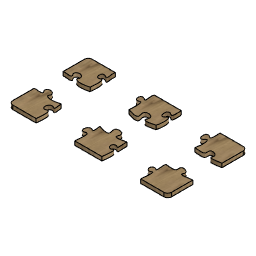
Púslu bretti v2 (Autodesk Fusion 360 design; units mm, degrees)
Autodesk Fusion 360 part; units mm, degrees
sketch "Sketch1" plane through (0, 0, 0) normal (0, 0, 1) x (1, 0, 0)
  line L0 (20, 0) -> (400, 0)
  line L1 (0, 240) -> (0, 20)
  line L2 (400, 260) -> (280, 260)
  line L3 (280, 260) -> (140, 260)
  line L4 (140, 260) -> (20, 260)
  line L5 (420, 240) -> (420, 130)
  line L6 (420, 130) -> (420, 20)
  spline S0 degree 5 poles (420, 130) (416.1569, 129.3347) (408.8145, 128.1) (398.8326, 126.5354) (387.5903, 125.0254) (376.9641, 124.1005) (369.6712, 124.1345) (365.4953, 125.1121) (364.0482, 127) (364.7182, 129.7413) (366.62, 133.2478) (368.5346, 137.3946) (369.2158, 141.9958) (367.694, 146.7817) (363.6047, 151.3716) (357.4467, 155.2591) (350.2289, 157.9216) (343.1844, 158.915) (337.448, 157.9813) (333.7805, 155.1362) (332.1898, 150.8086) (332.0622, 145.7217) (332.5096, 140.6598) (332.6186, 136.2944) (331.8011, 132.9328) (329.8033, 130.5545) (326.5513, 128.9847) (322.0312, 128.048) (316.2309, 127.6288) (309.1523, 127.6444) (300.8011, 128.0454) (293.1087, 128.653) (286.7739, 129.2656) (282.2998, 129.7436) (280, 130) knots 0 0 0 0 0 0 0.033333 0.066667 0.1 0.133333 0.166667 0.2 0.233333 0.266667 0.3 0.333333 0.366667 0.4 0.433333 0.466667 0.5 0.533333 0.566667 0.6 0.633333 0.666667 0.7 0.733333 0.766667 0.8 0.833333 0.866667 0.9 0.933333 0.966667 1 1 1 1 1 1
  spline S1 degree 5 poles (280, 130) (275.8224, 128.8825) (267.8961, 126.843) (257.2935, 124.3707) (245.7371, 122.2512) (235.5527, 121.5576) (229.4432, 122.7719) (226.9787, 125.7728) (227.3955, 130.3359) (229.4779, 136.0973) (231.5057, 142.5292) (231.7666, 149.0092) (228.9911, 154.8796) (222.8666, 159.5099) (214.3976, 162.358) (205.2875, 163.0238) (197.4083, 161.3087) (192.2863, 157.2675) (190.4715, 151.2893) (191.3079, 144.0924) (193.4639, 136.556) (195.2859, 129.5898) (195.2199, 123.9891) (192.1984, 120.2965) (185.5461, 118.8526) (174.8886, 119.8432) (163.0301, 122.6449) (152.2476, 125.8819) (144.2221, 128.5434) (140, 130) knots 0 0 0 0 0 0 0.04 0.08 0.12 0.16 0.2 0.24 0.28 0.32 0.36 0.4 0.44 0.48 0.52 0.56 0.6 0.64 0.68 0.72 0.76 0.8 0.84 0.88 0.92 0.96 1 1 1 1 1 1
  spline S2 degree 5 poles (0, 130) (0.6726, 130.1303) (2.0368, 130.3625) (4.1406, 130.6262) (7.0605, 130.808) (10.8974, 130.7621) (14.9065, 130.4737) (19.0576, 130.005) (23.2997, 129.4607) (27.5558, 128.9989) (31.712, 128.7955) (35.6093, 129.0115) (39.0309, 129.7574) (41.6968, 131.0621) (43.242, 132.8313) (43.385, 134.9274) (42.1144, 137.2617) (39.8723, 139.8827) (37.3749, 142.897) (35.4219, 146.3814) (34.7244, 150.3097) (35.6898, 154.4468) (38.3617, 158.3555) (42.5273, 161.5252) (47.7801, 163.4671) (53.6005, 163.8256) (59.4268, 162.4764) (64.7331, 159.6498) (69.0714, 155.8267) (72.1104, 151.6033) (73.6742, 147.5681) (73.7844, 144.1721) (72.6966, 141.607) (70.9513, 139.6629) (69.2082, 137.9334) (68.0891, 136.0141) (67.978, 133.7535) (69.0147, 131.2602) (71.2092, 128.7604) (74.5314, 126.4828) (78.963, 124.5976) (84.4839, 123.2388) (91.078, 122.5032) (98.7311, 122.4588) (107.4319, 123.1487) (117.1713, 124.5977) (125.7887, 126.3726) (132.7145, 128.0513) (137.5372, 129.3247) (140, 130) knots 0 0 0 0 0 0 0.022222 0.044444 0.066667 0.088889 0.111111 0.133333 0.155556 0.177778 0.2 0.222222 0.244444 0.266667 0.288889 0.311111 0.333333 0.355556 0.377778 0.4 0.422222 0.444444 0.466667 0.488889 0.511111 0.533333 0.555556 0.577778 0.6 0.622222 0.644444 0.666667 0.688889 0.711111 0.733333 0.755556 0.777778 0.8 0.822222 0.844444 0.866667 0.888889 0.911111 0.933333 0.955556 0.977778 1 1 1 1 1 1
  spline S3 degree 5 poles (280, 260) (280.191, 256.8907) (280.5235, 250.9394) (280.8735, 242.8142) (281.042, 233.5862) (280.7527, 224.7165) (279.9574, 218.457) (278.6472, 214.6822) (276.8095, 213.1654) (274.4294, 213.5546) (271.4855, 215.3325) (267.9643, 217.8215) (263.9195, 220.2718) (259.5123, 221.9338) (255.0824, 222.1325) (251.1161, 220.3585) (248.107, 216.3963) (246.4574, 210.4182) (246.3361, 203.1543) (247.6759, 195.7591) (250.2541, 189.4958) (253.7478, 185.4653) (257.7961, 184.3396) (262.0648, 186.0375) (266.2937, 189.5848) (270.2827, 193.5755) (273.8891, 196.5474) (277.02, 197.3547) (279.6286, 195.6325) (281.7019, 191.6447) (283.2467, 185.9595) (284.276, 179.1424) (284.7999, 171.5914) (284.8281, 163.5991) (284.3685, 155.3565) (283.4276, 146.9795) (282.2934, 140.2164) (281.2296, 135.1183) (280.4256, 131.708) (280, 130) knots 0 0 0 0 0 0 0.028571 0.057143 0.085714 0.114286 0.142857 0.171429 0.2 0.228571 0.257143 0.285714 0.314286 0.342857 0.371429 0.4 0.428571 0.457143 0.485714 0.514286 0.542857 0.571429 0.6 0.628571 0.657143 0.685714 0.714286 0.742857 0.771429 0.8 0.828571 0.857143 0.885714 0.914286 0.942857 0.971429 1 1 1 1 1 1
  spline S4 degree 5 poles (280, 130) (279.893, 129.6992) (279.7025, 128.9631) (279.4868, 127.4558) (279.3397, 124.6386) (279.3831, 119.8124) (279.631, 113.8173) (280.0368, 106.9315) (280.5206, 99.6325) (280.9623, 92.629) (281.2121, 86.6861) (281.0987, 82.4762) (280.4373, 80.4102) (279.042, 80.4986) (276.723, 82.1374) (273.3748, 84.3371) (269.0681, 86.0447) (264.1813, 86.486) (259.365, 85.297) (255.346, 82.4331) (252.7746, 78.1432) (252.058, 72.9178) (253.1887, 67.4537) (255.8568, 62.513) (259.5736, 58.7828) (263.7905, 56.7322) (268.0188, 56.4712) (271.9496, 57.6043) (275.4114, 59.408) (278.3264, 61.0095) (280.6676, 61.564) (282.4165, 60.431) (283.562, 57.1434) (284.0982, 51.3798) (284.0237, 42.937) (283.3393, 31.7027) (282.306, 20.4445) (281.2587, 10.7197) (280.4397, 3.668) (280, 0) knots 0 0 0 0 0 0 0.028571 0.057143 0.085714 0.114286 0.142857 0.171429 0.2 0.228571 0.257143 0.285714 0.314286 0.342857 0.371429 0.4 0.428571 0.457143 0.485714 0.514286 0.542857 0.571429 0.6 0.628571 0.657143 0.685714 0.714286 0.742857 0.771429 0.8 0.828571 0.857143 0.885714 0.914286 0.942857 0.971429 1 1 1 1 1 1
  spline S5 degree 5 poles (140, 260) (139.786, 259.149) (139.3949, 257.4189) (138.9194, 254.7391) (138.5076, 250.9966) (138.3554, 246.0496) (138.5404, 240.8764) (139.0108, 235.562) (139.6777, 230.2517) (140.4088, 225.1603) (141.0118, 220.6004) (141.2554, 216.9394) (140.9216, 214.4967) (139.8454, 213.4649) (137.9674, 213.805) (135.3596, 215.2012) (132.1765, 217.1928) (128.6213, 219.2678) (124.9018, 220.9885) (121.2137, 222.0296) (117.7406, 222.1651) (114.6502, 221.2708) (112.0908, 219.3206) (110.188, 216.3856) (109.039, 212.6276) (108.7059, 208.2939) (109.21, 203.7089) (110.5242, 199.275) (112.5703, 195.4454) (115.2295, 192.6298) (118.3503, 191.1054) (121.7572, 190.9403) (125.2582, 191.8765) (128.6582, 193.3586) (131.7822, 194.721) (134.4936, 195.3279) (136.7176, 194.743) (138.4568, 192.857) (139.7601, 189.7597) (140.6986, 185.6454) (141.3343, 180.6897) (141.7144, 175.0249) (141.8752, 168.7528) (141.8426, 161.9461) (141.6342, 154.6547) (141.261, 146.9088) (140.8351, 140.3614) (140.445, 135.2563) (140.1536, 131.7665) (140, 130) knots 0 0 0 0 0 0 0.022222 0.044444 0.066667 0.088889 0.111111 0.133333 0.155556 0.177778 0.2 0.222222 0.244444 0.266667 0.288889 0.311111 0.333333 0.355556 0.377778 0.4 0.422222 0.444444 0.466667 0.488889 0.511111 0.533333 0.555556 0.577778 0.6 0.622222 0.644444 0.666667 0.688889 0.711111 0.733333 0.755556 0.777778 0.8 0.822222 0.844444 0.866667 0.888889 0.911111 0.933333 0.955556 0.977778 1 1 1 1 1 1
  spline S6 degree 5 poles (140, 130) (140.3543, 127.5224) (141.0103, 122.7786) (141.836, 116.2971) (142.6203, 108.9248) (143.0716, 101.8141) (142.9936, 96.7592) (142.3884, 93.6536) (141.2613, 92.3088) (139.623, 92.4356) (137.4899, 93.6129) (134.8881, 95.293) (131.8674, 96.9199) (128.5115, 98.0179) (124.9543, 98.3121) (121.3675, 97.7073) (117.9388, 96.2219) (114.8545, 93.9421) (112.2772, 90.956) (110.3371, 87.3448) (109.1319, 83.2198) (108.7254, 78.7506) (109.1458, 74.1891) (110.3839, 69.9148) (112.3917, 66.3689) (115.0791, 63.9342) (118.3123, 62.8384) (121.9097, 63.0328) (125.6443, 64.1245) (129.2811, 65.5407) (132.6101, 66.6645) (135.4787, 66.9724) (137.8318, 66.1957) (139.6859, 64.2641) (141.0921, 61.2114) (142.0979, 57.0823) (142.7393, 51.9103) (143.0449, 45.725) (143.0355, 38.5494) (142.7258, 30.4016) (142.1253, 21.2949) (141.4167, 13.2494) (140.7578, 6.79) (140.262, 2.2948) (140, 0) knots 0 0 0 0 0 0 0.025 0.05 0.075 0.1 0.125 0.15 0.175 0.2 0.225 0.25 0.275 0.3 0.325 0.35 0.375 0.4 0.425 0.45 0.475 0.5 0.525 0.55 0.575 0.6 0.625 0.65 0.675 0.7 0.725 0.75 0.775 0.8 0.825 0.85 0.875 0.9 0.925 0.95 0.975 1 1 1 1 1 1
  arc A0 (420, 240) -> (400, 260) centre (400, 240) ccw
  arc A1 (400, 0) -> (420, 20) centre (400, 20) ccw
  arc A2 (0, 20) -> (20, 0) centre (20, 20) ccw
  arc A3 (20, 260) -> (0, 240) centre (20, 240) ccw
  line L7 (139.9962, -140.0866) -> (20, -140.0866)
  arc A4 (20, -140.0866) -> (0, -160.0866) centre (20, -160.0866) ccw
  line L8 (0, -160.0866) -> (0, -270)
  spline S7 degree 5 poles (139.9962, -140.0866) (139.7822, -140.9376) (139.3912, -142.6677) (138.9156, -145.3475) (138.5038, -149.09) (138.3517, -154.037) (138.5367, -159.2102) (139.007, -164.5246) (139.674, -169.8349) (140.4051, -174.9263) (141.0081, -179.4862) (141.2517, -183.1472) (140.9178, -185.5899) (139.8417, -186.6217) (137.9637, -186.2816) (135.3559, -184.8854) (132.1727, -182.8939) (128.6176, -180.8188) (124.8981, -179.0981) (121.2099, -178.057) (117.7369, -177.9215) (114.6465, -178.8158) (112.087, -180.7661) (110.1842, -183.701) (109.0352, -187.459) (108.7022, -191.7927) (109.2063, -196.3778) (110.5204, -200.8117) (112.5665, -204.6412) (115.2258, -207.4568) (118.3465, -208.9812) (121.7534, -209.1463) (125.2544, -208.2101) (128.6545, -206.728) (131.7784, -205.3656) (134.4898, -204.7587) (136.7138, -205.3436) (138.453, -207.2296) (139.7564, -210.3269) (140.6948, -214.4412) (141.3305, -219.3969) (141.7107, -225.0617) (141.8714, -231.3338) (141.8388, -238.1405) (141.6304, -245.4319) (141.2572, -253.1778) (140.8313, -259.7252) (140.4412, -264.8303) (140.1498, -268.3201) (139.9962, -270.0866) knots 0 0 0 0 0 0 0.022222 0.044444 0.066667 0.088889 0.111111 0.133333 0.155556 0.177778 0.2 0.222222 0.244444 0.266667 0.288889 0.311111 0.333333 0.355556 0.377778 0.4 0.422222 0.444444 0.466667 0.488889 0.511111 0.533333 0.555556 0.577778 0.6 0.622222 0.644444 0.666667 0.688889 0.711111 0.733333 0.755556 0.777778 0.8 0.822222 0.844444 0.866667 0.888889 0.911111 0.933333 0.955556 0.977778 1 1 1 1 1 1
  spline S8 degree 5 poles (0, -270) (0.6726, -269.8697) (2.0368, -269.6375) (4.1406, -269.3738) (7.0605, -269.192) (10.8973, -269.2379) (14.9064, -269.5263) (19.0574, -269.995) (23.2996, -270.5393) (27.5556, -271.0011) (31.7119, -271.2045) (35.6091, -270.9885) (39.0307, -270.2426) (41.6966, -268.938) (43.242, -267.1689) (43.3851, -265.0728) (42.1146, -262.7385) (39.8725, -260.1175) (37.3751, -257.1032) (35.422, -253.6189) (34.7243, -249.6907) (35.6896, -245.5537) (38.3613, -241.645) (42.5267, -238.4752) (47.7794, -236.5331) (53.5997, -236.1743) (59.426, -237.5232) (64.7324, -240.3495) (69.0709, -244.1724) (72.11, -248.3958) (73.674, -252.4311) (73.7845, -255.8274) (72.6969, -258.3928) (70.9516, -260.3371) (69.2085, -262.0664) (68.0892, -263.9853) (67.9779, -266.2455) (69.0144, -268.7388) (71.2086, -271.2394) (74.5306, -273.519) (78.9619, -275.4078) (84.4824, -276.7719) (91.0762, -277.5148) (98.7291, -277.5686) (107.4294, -276.8901) (117.1684, -275.4547) (125.7854, -273.6924) (132.711, -272.0241) (137.5336, -270.7581) (139.9962, -270.0866) knots 0 0 0 0 0 0 0.022222 0.044444 0.066667 0.088889 0.111111 0.133333 0.155556 0.177778 0.2 0.222222 0.244444 0.266667 0.288889 0.311111 0.333333 0.355556 0.377778 0.4 0.422222 0.444444 0.466667 0.488889 0.511111 0.533333 0.555556 0.577778 0.6 0.622222 0.644444 0.666667 0.688889 0.711111 0.733333 0.755556 0.777778 0.8 0.822222 0.844444 0.866667 0.888889 0.911111 0.933333 0.955556 0.977778 1 1 1 1 1 1
  spline S9 degree 5 poles (140, -420) (140.3543, -422.4776) (141.0103, -427.2214) (141.836, -433.7029) (142.6203, -441.0752) (143.0716, -448.1859) (142.9936, -453.2408) (142.3884, -456.3464) (141.2613, -457.6912) (139.623, -457.5644) (137.4899, -456.3871) (134.8881, -454.707) (131.8674, -453.0801) (128.5115, -451.9821) (124.9543, -451.6879) (121.3675, -452.2927) (117.9388, -453.7781) (114.8545, -456.0579) (112.2772, -459.044) (110.3371, -462.6552) (109.1319, -466.7802) (108.7254, -471.2494) (109.1458, -475.8109) (110.3839, -480.0852) (112.3917, -483.6311) (115.0791, -486.0658) (118.3123, -487.1616) (121.9097, -486.9672) (125.6443, -485.8755) (129.2811, -484.4593) (132.6101, -483.3355) (135.4787, -483.0276) (137.8318, -483.8043) (139.6859, -485.7359) (141.0921, -488.7886) (142.0979, -492.9177) (142.7393, -498.0897) (143.0449, -504.275) (143.0355, -511.4506) (142.7258, -519.5984) (142.1253, -528.7051) (141.4167, -536.7506) (140.7578, -543.21) (140.262, -547.7052) (140, -550) knots 0 0 0 0 0 0 0.025 0.05 0.075 0.1 0.125 0.15 0.175 0.2 0.225 0.25 0.275 0.3 0.325 0.35 0.375 0.4 0.425 0.45 0.475 0.5 0.525 0.55 0.575 0.6 0.625 0.65 0.675 0.7 0.725 0.75 0.775 0.8 0.825 0.85 0.875 0.9 0.925 0.95 0.975 1 1 1 1 1 1
  spline S10 degree 5 poles (0, -420) (0.6726, -419.8697) (2.0368, -419.6375) (4.1406, -419.3738) (7.0605, -419.192) (10.8974, -419.2379) (14.9065, -419.5263) (19.0576, -419.995) (23.2997, -420.5393) (27.5558, -421.0011) (31.712, -421.2045) (35.6093, -420.9885) (39.0309, -420.2426) (41.6968, -418.9379) (43.242, -417.1687) (43.385, -415.0726) (42.1144, -412.7383) (39.8723, -410.1173) (37.3749, -407.103) (35.4219, -403.6186) (34.7244, -399.6903) (35.6898, -395.5532) (38.3617, -391.6445) (42.5273, -388.4748) (47.7801, -386.5329) (53.6005, -386.1744) (59.4268, -387.5236) (64.7331, -390.3502) (69.0714, -394.1733) (72.1104, -398.3968) (73.6742, -402.4319) (73.7844, -405.8279) (72.6966, -408.393) (70.9513, -410.3371) (69.2082, -412.0666) (68.0891, -413.9859) (67.978, -416.2465) (69.0147, -418.7398) (71.2092, -421.2396) (74.5314, -423.5172) (78.963, -425.4024) (84.4839, -426.7612) (91.078, -427.4968) (98.7311, -427.5412) (107.4319, -426.8513) (117.1713, -425.4023) (125.7887, -423.6274) (132.7145, -421.9487) (137.5372, -420.6753) (140, -420) knots 0 0 0 0 0 0 0.022222 0.044444 0.066667 0.088889 0.111111 0.133333 0.155556 0.177778 0.2 0.222222 0.244444 0.266667 0.288889 0.311111 0.333333 0.355556 0.377778 0.4 0.422222 0.444444 0.466667 0.488889 0.511111 0.533333 0.555556 0.577778 0.6 0.622222 0.644444 0.666667 0.688889 0.711111 0.733333 0.755556 0.777778 0.8 0.822222 0.844444 0.866667 0.888889 0.911111 0.933333 0.955556 0.977778 1 1 1 1 1 1
  line L9 (0, -420) -> (0, -530)
  arc A5 (0, -530) -> (20, -550) centre (20, -530) ccw
  line L10 (20, -550) -> (140, -550)
  spline S11 degree 5 poles (140, 130) (140.3543, 127.5224) (141.0103, 122.7786) (141.836, 116.2971) (142.6203, 108.9248) (143.0716, 101.8141) (142.9936, 96.7592) (142.3884, 93.6536) (141.2613, 92.3088) (139.623, 92.4356) (137.4899, 93.6129) (134.8881, 95.293) (131.8674, 96.9199) (128.5115, 98.0179) (124.9543, 98.3121) (121.3675, 97.7073) (117.9388, 96.2219) (114.8545, 93.9421) (112.2772, 90.956) (110.3371, 87.3448) (109.1319, 83.2198) (108.7254, 78.7506) (109.1458, 74.1891) (110.3839, 69.9148) (112.3917, 66.3689) (115.0791, 63.9342) (118.3123, 62.8384) (121.9097, 63.0328) (125.6443, 64.1245) (129.2811, 65.5407) (132.6101, 66.6645) (135.4787, 66.9724) (137.8318, 66.1957) (139.6859, 64.2641) (141.0921, 61.2114) (142.0979, 57.0823) (142.7393, 51.9103) (143.0449, 45.725) (143.0355, 38.5494) (142.7258, 30.4016) (142.1253, 21.2949) (141.4167, 13.2494) (140.7578, 6.79) (140.262, 2.2948) (140, 0) knots 0 0 0 0 0 0 0.025 0.05 0.075 0.1 0.125 0.15 0.175 0.2 0.225 0.25 0.275 0.3 0.325 0.35 0.375 0.4 0.425 0.45 0.475 0.5 0.525 0.55 0.575 0.6 0.625 0.65 0.675 0.7 0.725 0.75 0.775 0.8 0.825 0.85 0.875 0.9 0.925 0.95 0.975 1 1 1 1 1 1
  spline S12 degree 5 poles (280, 130) (275.8224, 128.8825) (267.8961, 126.843) (257.2935, 124.3707) (245.7371, 122.2512) (235.5527, 121.5576) (229.4432, 122.7719) (226.9787, 125.7728) (227.3955, 130.3359) (229.4779, 136.0973) (231.5057, 142.5292) (231.7666, 149.0092) (228.9911, 154.8796) (222.8666, 159.5099) (214.3976, 162.358) (205.2875, 163.0238) (197.4083, 161.3087) (192.2863, 157.2675) (190.4715, 151.2893) (191.3079, 144.0924) (193.4639, 136.556) (195.2859, 129.5898) (195.2199, 123.9891) (192.1984, 120.2965) (185.5461, 118.8526) (174.8886, 119.8432) (163.0301, 122.6449) (152.2476, 125.8819) (144.2221, 128.5434) (140, 130) knots 0 0 0 0 0 0 0.04 0.08 0.12 0.16 0.2 0.24 0.28 0.32 0.36 0.4 0.44 0.48 0.52 0.56 0.6 0.64 0.68 0.72 0.76 0.8 0.84 0.88 0.92 0.96 1 1 1 1 1 1
  line L11 (20, 0) -> (400, 0)
  spline S13 degree 5 poles (280, 130) (279.893, 129.6992) (279.7025, 128.9631) (279.4868, 127.4558) (279.3397, 124.6386) (279.3831, 119.8124) (279.631, 113.8173) (280.0368, 106.9315) (280.5206, 99.6325) (280.9623, 92.629) (281.2121, 86.6861) (281.0987, 82.4762) (280.4373, 80.4102) (279.042, 80.4986) (276.723, 82.1374) (273.3748, 84.3371) (269.0681, 86.0447) (264.1813, 86.486) (259.365, 85.297) (255.346, 82.4331) (252.7746, 78.1432) (252.058, 72.9178) (253.1887, 67.4537) (255.8568, 62.513) (259.5736, 58.7828) (263.7905, 56.7322) (268.0188, 56.4712) (271.9496, 57.6043) (275.4114, 59.408) (278.3264, 61.0095) (280.6676, 61.564) (282.4165, 60.431) (283.562, 57.1434) (284.0982, 51.3798) (284.0237, 42.937) (283.3393, 31.7027) (282.306, 20.4445) (281.2587, 10.7197) (280.4397, 3.668) (280, 0) knots 0 0 0 0 0 0 0.028571 0.057143 0.085714 0.114286 0.142857 0.171429 0.2 0.228571 0.257143 0.285714 0.314286 0.342857 0.371429 0.4 0.428571 0.457143 0.485714 0.514286 0.542857 0.571429 0.6 0.628571 0.657143 0.685714 0.714286 0.742857 0.771429 0.8 0.828571 0.857143 0.885714 0.914286 0.942857 0.971429 1 1 1 1 1 1
  line L12 (20, 0) -> (400, 0)
  spline S14 degree 5 poles (280, 130) (275.8224, 128.8825) (267.8961, 126.843) (257.2935, 124.3707) (245.7371, 122.2512) (235.5527, 121.5576) (229.4432, 122.7719) (226.9787, 125.7728) (227.3955, 130.3359) (229.4779, 136.0973) (231.5057, 142.5292) (231.7666, 149.0092) (228.9911, 154.8796) (222.8666, 159.5099) (214.3976, 162.358) (205.2875, 163.0238) (197.4083, 161.3087) (192.2863, 157.2675) (190.4715, 151.2893) (191.3079, 144.0924) (193.4639, 136.556) (195.2859, 129.5898) (195.2199, 123.9891) (192.1984, 120.2965) (185.5461, 118.8526) (174.8886, 119.8432) (163.0301, 122.6449) (152.2476, 125.8819) (144.2221, 128.5434) (140, 130) knots 0 0 0 0 0 0 0.04 0.08 0.12 0.16 0.2 0.24 0.28 0.32 0.36 0.4 0.44 0.48 0.52 0.56 0.6 0.64 0.68 0.72 0.76 0.8 0.84 0.88 0.92 0.96 1 1 1 1 1 1
  spline S15 degree 5 poles (140, 130) (140.3543, 127.5224) (141.0103, 122.7786) (141.836, 116.2971) (142.6203, 108.9248) (143.0716, 101.8141) (142.9936, 96.7592) (142.3884, 93.6536) (141.2613, 92.3088) (139.623, 92.4356) (137.4899, 93.6129) (134.8881, 95.293) (131.8674, 96.9199) (128.5115, 98.0179) (124.9543, 98.3121) (121.3675, 97.7073) (117.9388, 96.2219) (114.8545, 93.9421) (112.2772, 90.956) (110.3371, 87.3448) (109.1319, 83.2198) (108.7254, 78.7506) (109.1458, 74.1891) (110.3839, 69.9148) (112.3917, 66.3689) (115.0791, 63.9342) (118.3123, 62.8384) (121.9097, 63.0328) (125.6443, 64.1245) (129.2811, 65.5407) (132.6101, 66.6645) (135.4787, 66.9724) (137.8318, 66.1957) (139.6859, 64.2641) (141.0921, 61.2114) (142.0979, 57.0823) (142.7393, 51.9103) (143.0449, 45.725) (143.0355, 38.5494) (142.7258, 30.4016) (142.1253, 21.2949) (141.4167, 13.2494) (140.7578, 6.79) (140.262, 2.2948) (140, 0) knots 0 0 0 0 0 0 0.025 0.05 0.075 0.1 0.125 0.15 0.175 0.2 0.225 0.25 0.275 0.3 0.325 0.35 0.375 0.4 0.425 0.45 0.475 0.5 0.525 0.55 0.575 0.6 0.625 0.65 0.675 0.7 0.725 0.75 0.775 0.8 0.825 0.85 0.875 0.9 0.925 0.95 0.975 1 1 1 1 1 1
  line L13 (340, -550) -> (480, -550)
  spline S16 degree 5 poles (480, -420) (479.893, -420.3008) (479.7025, -421.0369) (479.4868, -422.5442) (479.3397, -425.3614) (479.3831, -430.1876) (479.631, -436.1827) (480.0368, -443.0685) (480.5206, -450.3675) (480.9623, -457.371) (481.2121, -463.3139) (481.0987, -467.5238) (480.4373, -469.5898) (479.042, -469.5014) (476.723, -467.8626) (473.3748, -465.6629) (469.0681, -463.9553) (464.1813, -463.514) (459.365, -464.703) (455.346, -467.5669) (452.7746, -471.8568) (452.058, -477.0822) (453.1887, -482.5463) (455.8568, -487.487) (459.5736, -491.2172) (463.7905, -493.2678) (468.0188, -493.5288) (471.9496, -492.3957) (475.4114, -490.592) (478.3264, -488.9905) (480.6676, -488.436) (482.4165, -489.569) (483.562, -492.8566) (484.0982, -498.6202) (484.0237, -507.063) (483.3393, -518.2973) (482.306, -529.5555) (481.2587, -539.2803) (480.4397, -546.332) (480, -550) knots 0 0 0 0 0 0 0.028571 0.057143 0.085714 0.114286 0.142857 0.171429 0.2 0.228571 0.257143 0.285714 0.314286 0.342857 0.371429 0.4 0.428571 0.457143 0.485714 0.514286 0.542857 0.571429 0.6 0.628571 0.657143 0.685714 0.714286 0.742857 0.771429 0.8 0.828571 0.857143 0.885714 0.914286 0.942857 0.971429 1 1 1 1 1 1
  spline S17 degree 5 poles (480, -420) (475.8224, -421.1175) (467.8961, -423.157) (457.2935, -425.6293) (445.7371, -427.7488) (435.5527, -428.4424) (429.4432, -427.2281) (426.9787, -424.2272) (427.3955, -419.6641) (429.4779, -413.9027) (431.5057, -407.4708) (431.7666, -400.9908) (428.9911, -395.1204) (422.8666, -390.4901) (414.3976, -387.642) (405.2875, -386.9762) (397.4083, -388.6913) (392.2863, -392.7325) (390.4715, -398.7107) (391.3079, -405.9076) (393.4639, -413.444) (395.2859, -420.4102) (395.2199, -426.0109) (392.1984, -429.7035) (385.5461, -431.1474) (374.8886, -430.1568) (363.0301, -427.3551) (352.2476, -424.1181) (344.2221, -421.4566) (340, -420) knots 0 0 0 0 0 0 0.04 0.08 0.12 0.16 0.2 0.24 0.28 0.32 0.36 0.4 0.44 0.48 0.52 0.56 0.6 0.64 0.68 0.72 0.76 0.8 0.84 0.88 0.92 0.96 1 1 1 1 1 1
  spline S18 degree 5 poles (340, -420) (340.3543, -422.4776) (341.0103, -427.2214) (341.836, -433.7029) (342.6203, -441.0752) (343.0716, -448.1859) (342.9936, -453.2408) (342.3884, -456.3464) (341.2613, -457.6912) (339.623, -457.5644) (337.4899, -456.3871) (334.8881, -454.707) (331.8674, -453.0801) (328.5115, -451.9821) (324.9543, -451.6879) (321.3675, -452.2927) (317.9388, -453.7781) (314.8545, -456.0579) (312.2772, -459.044) (310.3371, -462.6552) (309.1319, -466.7802) (308.7254, -471.2494) (309.1458, -475.8109) (310.3839, -480.0852) (312.3917, -483.6311) (315.0791, -486.0658) (318.3123, -487.1616) (321.9097, -486.9672) (325.6443, -485.8755) (329.2811, -484.4593) (332.6101, -483.3355) (335.4787, -483.0276) (337.8318, -483.8043) (339.6859, -485.7359) (341.0921, -488.7886) (342.0979, -492.9177) (342.7393, -498.0897) (343.0449, -504.275) (343.0355, -511.4506) (342.7258, -519.5984) (342.1253, -528.7051) (341.4167, -536.7506) (340.7578, -543.21) (340.262, -547.7052) (340, -550) knots 0 0 0 0 0 0 0.025 0.05 0.075 0.1 0.125 0.15 0.175 0.2 0.225 0.25 0.275 0.3 0.325 0.35 0.375 0.4 0.425 0.45 0.475 0.5 0.525 0.55 0.575 0.6 0.625 0.65 0.675 0.7 0.725 0.75 0.775 0.8 0.825 0.85 0.875 0.9 0.925 0.95 0.975 1 1 1 1 1 1
  spline S19 degree 5 poles (480, -140) (480.191, -143.1093) (480.5235, -149.0606) (480.8735, -157.1858) (481.042, -166.4138) (480.7527, -175.2835) (479.9574, -181.543) (478.6472, -185.3178) (476.8095, -186.8346) (474.4294, -186.4454) (471.4855, -184.6675) (467.9643, -182.1785) (463.9195, -179.7282) (459.5123, -178.0662) (455.0824, -177.8675) (451.1161, -179.6415) (448.107, -183.6037) (446.4574, -189.5818) (446.3361, -196.8457) (447.6759, -204.2409) (450.2541, -210.5042) (453.7478, -214.5347) (457.7961, -215.6604) (462.0648, -213.9625) (466.2937, -210.4152) (470.2827, -206.4245) (473.8891, -203.4526) (477.02, -202.6453) (479.6286, -204.3675) (481.7019, -208.3553) (483.2467, -214.0405) (484.276, -220.8576) (484.7999, -228.4086) (484.8281, -236.4009) (484.3685, -244.6435) (483.4276, -253.0205) (482.2934, -259.7836) (481.2296, -264.8817) (480.4256, -268.292) (480, -270) knots 0 0 0 0 0 0 0.028571 0.057143 0.085714 0.114286 0.142857 0.171429 0.2 0.228571 0.257143 0.285714 0.314286 0.342857 0.371429 0.4 0.428571 0.457143 0.485714 0.514286 0.542857 0.571429 0.6 0.628571 0.657143 0.685714 0.714286 0.742857 0.771429 0.8 0.828571 0.857143 0.885714 0.914286 0.942857 0.971429 1 1 1 1 1 1
  line L14 (480, -140) -> (340, -140)
  spline S20 degree 5 poles (340, -140) (339.786, -140.851) (339.3949, -142.5811) (338.9194, -145.2609) (338.5076, -149.0034) (338.3554, -153.9504) (338.5404, -159.1236) (339.0108, -164.438) (339.6777, -169.7483) (340.4088, -174.8397) (341.0118, -179.3996) (341.2554, -183.0606) (340.9216, -185.5033) (339.8454, -186.5351) (337.9674, -186.195) (335.3596, -184.7988) (332.1765, -182.8072) (328.6213, -180.7322) (324.9018, -179.0115) (321.2137, -177.9704) (317.7406, -177.8349) (314.6502, -178.7292) (312.0908, -180.6794) (310.188, -183.6144) (309.039, -187.3724) (308.7059, -191.7061) (309.21, -196.2911) (310.5242, -200.725) (312.5703, -204.5546) (315.2295, -207.3702) (318.3503, -208.8946) (321.7572, -209.0597) (325.2582, -208.1235) (328.6582, -206.6414) (331.7822, -205.279) (334.4936, -204.6721) (336.7176, -205.257) (338.4568, -207.143) (339.7601, -210.2403) (340.6986, -214.3546) (341.3343, -219.3103) (341.7144, -224.9751) (341.8752, -231.2472) (341.8426, -238.0539) (341.6342, -245.3453) (341.261, -253.0912) (340.8351, -259.6386) (340.445, -264.7437) (340.1536, -268.2335) (340, -270) knots 0 0 0 0 0 0 0.022222 0.044444 0.066667 0.088889 0.111111 0.133333 0.155556 0.177778 0.2 0.222222 0.244444 0.266667 0.288889 0.311111 0.333333 0.355556 0.377778 0.4 0.422222 0.444444 0.466667 0.488889 0.511111 0.533333 0.555556 0.577778 0.6 0.622222 0.644444 0.666667 0.688889 0.711111 0.733333 0.755556 0.777778 0.8 0.822222 0.844444 0.866667 0.888889 0.911111 0.933333 0.955556 0.977778 1 1 1 1 1 1
  spline S21 degree 5 poles (480, -270) (475.8224, -271.1175) (467.8961, -273.157) (457.2935, -275.6293) (445.7371, -277.7488) (435.5527, -278.4424) (429.4432, -277.2281) (426.9787, -274.2272) (427.3955, -269.6641) (429.4779, -263.9027) (431.5057, -257.4708) (431.7666, -250.9908) (428.9911, -245.1204) (422.8666, -240.4901) (414.3976, -237.642) (405.2875, -236.9762) (397.4083, -238.6913) (392.2863, -242.7325) (390.4715, -248.7107) (391.3079, -255.9076) (393.4639, -263.444) (395.2859, -270.4102) (395.2199, -276.0109) (392.1984, -279.7035) (385.5461, -281.1474) (374.8886, -280.1568) (363.0301, -277.3551) (352.2476, -274.1181) (344.2221, -271.4566) (340, -270) knots 0 0 0 0 0 0 0.04 0.08 0.12 0.16 0.2 0.24 0.28 0.32 0.36 0.4 0.44 0.48 0.52 0.56 0.6 0.64 0.68 0.72 0.76 0.8 0.84 0.88 0.92 0.96 1 1 1 1 1 1
  line L15 (400, 260) -> (280, 260)
  spline S22 degree 5 poles (280, 260) (280.191, 256.8907) (280.5235, 250.9394) (280.8735, 242.8142) (281.042, 233.5862) (280.7527, 224.7165) (279.9574, 218.457) (278.6472, 214.6822) (276.8095, 213.1654) (274.4294, 213.5546) (271.4855, 215.3325) (267.9643, 217.8215) (263.9195, 220.2718) (259.5123, 221.9338) (255.0824, 222.1325) (251.1161, 220.3585) (248.107, 216.3963) (246.4574, 210.4182) (246.3361, 203.1543) (247.6759, 195.7591) (250.2541, 189.4958) (253.7478, 185.4653) (257.7961, 184.3396) (262.0648, 186.0375) (266.2937, 189.5848) (270.2827, 193.5755) (273.8891, 196.5474) (277.02, 197.3547) (279.6286, 195.6325) (281.7019, 191.6447) (283.2467, 185.9595) (284.276, 179.1424) (284.7999, 171.5914) (284.8281, 163.5991) (284.3685, 155.3565) (283.4276, 146.9795) (282.2934, 140.2164) (281.2296, 135.1183) (280.4256, 131.708) (280, 130) knots 0 0 0 0 0 0 0.028571 0.057143 0.085714 0.114286 0.142857 0.171429 0.2 0.228571 0.257143 0.285714 0.314286 0.342857 0.371429 0.4 0.428571 0.457143 0.485714 0.514286 0.542857 0.571429 0.6 0.628571 0.657143 0.685714 0.714286 0.742857 0.771429 0.8 0.828571 0.857143 0.885714 0.914286 0.942857 0.971429 1 1 1 1 1 1
  spline S23 degree 5 poles (420, 130) (416.1569, 129.3347) (408.8145, 128.1) (398.8326, 126.5354) (387.5903, 125.0254) (376.9641, 124.1005) (369.6712, 124.1345) (365.4953, 125.1121) (364.0482, 127) (364.7182, 129.7413) (366.62, 133.2478) (368.5346, 137.3946) (369.2158, 141.9958) (367.694, 146.7817) (363.6047, 151.3716) (357.4467, 155.2591) (350.2289, 157.9216) (343.1844, 158.915) (337.448, 157.9813) (333.7805, 155.1362) (332.1898, 150.8086) (332.0622, 145.7217) (332.5096, 140.6598) (332.6186, 136.2944) (331.8011, 132.9328) (329.8033, 130.5545) (326.5513, 128.9847) (322.0312, 128.048) (316.2309, 127.6288) (309.1523, 127.6444) (300.8011, 128.0454) (293.1087, 128.653) (286.7739, 129.2656) (282.2998, 129.7436) (280, 130) knots 0 0 0 0 0 0 0.033333 0.066667 0.1 0.133333 0.166667 0.2 0.233333 0.266667 0.3 0.333333 0.366667 0.4 0.433333 0.466667 0.5 0.533333 0.566667 0.6 0.633333 0.666667 0.7 0.733333 0.766667 0.8 0.833333 0.866667 0.9 0.933333 0.966667 1 1 1 1 1 1
  line L16 (420, 240) -> (420, 130)
  arc A6 (820, -160) -> (800, -140) centre (800, -160) ccw
  line L17 (820, -160) -> (820, -270)
  spline S24 degree 5 poles (820, -270) (816.1569, -270.6653) (808.8145, -271.9) (798.8326, -273.4646) (787.5903, -274.9746) (776.9641, -275.8995) (769.6712, -275.8655) (765.4953, -274.8879) (764.0482, -273) (764.7182, -270.2587) (766.62, -266.7522) (768.5346, -262.6054) (769.2158, -258.0042) (767.694, -253.2183) (763.6047, -248.6284) (757.4467, -244.7409) (750.2289, -242.0784) (743.1844, -241.085) (737.448, -242.0187) (733.7805, -244.8638) (732.1898, -249.1914) (732.0622, -254.2783) (732.5096, -259.3402) (732.6186, -263.7056) (731.8011, -267.0672) (729.8033, -269.4455) (726.5513, -271.0153) (722.0312, -271.952) (716.2309, -272.3712) (709.1523, -272.3556) (700.8011, -271.9546) (693.1087, -271.347) (686.7739, -270.7344) (682.2998, -270.2564) (680, -270) knots 0 0 0 0 0 0 0.033333 0.066667 0.1 0.133333 0.166667 0.2 0.233333 0.266667 0.3 0.333333 0.366667 0.4 0.433333 0.466667 0.5 0.533333 0.566667 0.6 0.633333 0.666667 0.7 0.733333 0.766667 0.8 0.833333 0.866667 0.9 0.933333 0.966667 1 1 1 1 1 1
  spline S25 degree 5 poles (680, -140) (680.191, -143.1093) (680.5235, -149.0606) (680.8735, -157.1858) (681.042, -166.4138) (680.7527, -175.2835) (679.9574, -181.543) (678.6472, -185.3178) (676.8095, -186.8346) (674.4294, -186.4454) (671.4855, -184.6675) (667.9643, -182.1785) (663.9195, -179.7282) (659.5123, -178.0662) (655.0824, -177.8675) (651.1161, -179.6415) (648.107, -183.6037) (646.4574, -189.5818) (646.3361, -196.8457) (647.6759, -204.2409) (650.2541, -210.5042) (653.7478, -214.5347) (657.7961, -215.6604) (662.0648, -213.9625) (666.2937, -210.4152) (670.2827, -206.4245) (673.8891, -203.4526) (677.02, -202.6453) (679.6286, -204.3675) (681.7019, -208.3553) (683.2467, -214.0405) (684.276, -220.8576) (684.7999, -228.4086) (684.8281, -236.4009) (684.3685, -244.6435) (683.4276, -253.0205) (682.2934, -259.7836) (681.2296, -264.8817) (680.4256, -268.292) (680, -270) knots 0 0 0 0 0 0 0.028571 0.057143 0.085714 0.114286 0.142857 0.171429 0.2 0.228571 0.257143 0.285714 0.314286 0.342857 0.371429 0.4 0.428571 0.457143 0.485714 0.514286 0.542857 0.571429 0.6 0.628571 0.657143 0.685714 0.714286 0.742857 0.771429 0.8 0.828571 0.857143 0.885714 0.914286 0.942857 0.971429 1 1 1 1 1 1
  line L18 (800, -140) -> (680, -140)
  arc A7 (800, -550) -> (820, -530) centre (800, -530) ccw
  line L19 (820, -420) -> (820, -530)
  spline S26 degree 5 poles (820, -420) (816.1569, -420.6653) (808.8145, -421.9) (798.8326, -423.4646) (787.5903, -424.9746) (776.9641, -425.8995) (769.6712, -425.8655) (765.4953, -424.8879) (764.0482, -423) (764.7182, -420.2587) (766.62, -416.7522) (768.5346, -412.6054) (769.2158, -408.0042) (767.694, -403.2183) (763.6047, -398.6284) (757.4467, -394.7409) (750.2289, -392.0784) (743.1844, -391.085) (737.448, -392.0187) (733.7805, -394.8638) (732.1898, -399.1914) (732.0622, -404.2783) (732.5096, -409.3402) (732.6186, -413.7056) (731.8011, -417.0672) (729.8033, -419.4455) (726.5513, -421.0153) (722.0312, -421.952) (716.2309, -422.3712) (709.1523, -422.3556) (700.8011, -421.9546) (693.1087, -421.347) (686.7739, -420.7344) (682.2998, -420.2564) (680, -420) knots 0 0 0 0 0 0 0.033333 0.066667 0.1 0.133333 0.166667 0.2 0.233333 0.266667 0.3 0.333333 0.366667 0.4 0.433333 0.466667 0.5 0.533333 0.566667 0.6 0.633333 0.666667 0.7 0.733333 0.766667 0.8 0.833333 0.866667 0.9 0.933333 0.966667 1 1 1 1 1 1
  spline S27 degree 5 poles (680, -420) (679.893, -420.3008) (679.7025, -421.0369) (679.4868, -422.5442) (679.3397, -425.3614) (679.3831, -430.1876) (679.631, -436.1827) (680.0368, -443.0685) (680.5206, -450.3675) (680.9623, -457.371) (681.2121, -463.3139) (681.0987, -467.5238) (680.4373, -469.5898) (679.042, -469.5014) (676.723, -467.8626) (673.3748, -465.6629) (669.0681, -463.9553) (664.1813, -463.514) (659.365, -464.703) (655.346, -467.5669) (652.7746, -471.8568) (652.058, -477.0822) (653.1887, -482.5463) (655.8568, -487.487) (659.5736, -491.2172) (663.7905, -493.2678) (668.0188, -493.5288) (671.9496, -492.3957) (675.4114, -490.592) (678.3264, -488.9905) (680.6676, -488.436) (682.4165, -489.569) (683.562, -492.8566) (684.0982, -498.6202) (684.0237, -507.063) (683.3393, -518.2973) (682.306, -529.5555) (681.2587, -539.2803) (680.4397, -546.332) (680, -550) knots 0 0 0 0 0 0 0.028571 0.057143 0.085714 0.114286 0.142857 0.171429 0.2 0.228571 0.257143 0.285714 0.314286 0.342857 0.371429 0.4 0.428571 0.457143 0.485714 0.514286 0.542857 0.571429 0.6 0.628571 0.657143 0.685714 0.714286 0.742857 0.771429 0.8 0.828571 0.857143 0.885714 0.914286 0.942857 0.971429 1 1 1 1 1 1
  line L20 (680, -550) -> (800, -550)
  spline S28 degree 3 poles (139.0265, -139.8427) (137.9907, -143.9604) (137.4767, -148.4646) (137.4379, -153.2806) (137.4019, -157.7485) (137.7867, -162.5045) (138.3482, -167.1553) (138.8747, -171.5155) (139.5573, -175.7899) (139.901, -179.1404) (140.0934, -181.0158) (140.1667, -182.5956) (140.0608, -183.6748) (139.9881, -184.4145) (139.8189, -184.8993) (139.6812, -185.1018) (139.5721, -185.2623) (139.5326, -185.2821) (139.3904, -185.313) (139.2048, -185.3533) (138.7604, -185.3185) (138.1209, -185.0779) (136.8139, -184.5862) (134.8202, -183.3382) (132.5658, -181.9979) (129.7891, -180.3472) (126.5895, -178.6168) (123.4366, -177.7405) (120.7368, -176.9901) (118.0479, -176.855) (115.6835, -177.6274) (113.3644, -178.3851) (111.4064, -180.0241) (110.078, -182.3009) (108.3637, -185.2388) (107.6569, -189.2322) (107.986, -193.3889) (108.3197, -197.6038) (109.7175, -201.9532) (111.9932, -205.0917) (113.4698, -207.1282) (115.3325, -208.6465) (117.4202, -209.3829) (119.357, -210.0662) (121.4494, -210.0513) (123.4553, -209.612) (125.8499, -209.0877) (128.1492, -208.0057) (130.1499, -207.1891) (131.7043, -206.5547) (133.0715, -206.1086) (134.1262, -206.0591) (135.1443, -206.0112) (135.8651, -206.2561) (136.5713, -206.9043) (137.4083, -207.6725) (138.1835, -209.1161) (138.7902, -211.139) (139.7571, -214.3633) (140.3251, -218.9337) (140.6084, -224.2788) (140.9575, -230.8659) (140.8895, -238.644) (140.5183, -247.2591) (140.2161, -254.2743) (139.7073, -261.863) (139, -270) knots 0 0 0 0 0.06311736 0.06311736 0.06311736 0.12167253 0.12167253 0.12167253 0.176568 0.176568 0.176568 0.20729468 0.20729468 0.20729468 0.22835242 0.22835242 0.22835242 0.24503512 0.24503512 0.24503512 0.26679691 0.26679691 0.26679691 0.31127682 0.31127682 0.31127682 0.36606173 0.36606173 0.36606173 0.41297316 0.41297316 0.41297316 0.45898499 0.45898499 0.45898499 0.51835872 0.51835872 0.51835872 0.57856388 0.57856388 0.57856388 0.61762929 0.61762929 0.61762929 0.65387232 0.65387232 0.65387232 0.69713828 0.69713828 0.69713828 0.73075322 0.73075322 0.73075322 0.76320073 0.76320073 0.76320073 0.80165605 0.80165605 0.80165605 0.86295163 0.86295163 0.86295163 0.93848985 0.93848985 0.93848985 1 1 1 1
  point P0 (420, 260)
  point P1 (0, 260)
  point P2 (365.0496, 130)
  point P3 (367.3759, 146.1756)
  point P4 (336.6686, 156.8767)
  point P5 (332.4813, 139.1967)
  point P6 (328.2939, 130)
  point P7 (227.6791, 130)
  point P8 (228.7481, 153.837)
  point P9 (194.5419, 158.4355)
  point P10 (194.8091, 130)
  point P11 (18.966, 130)
  point P12 (39.1362, 130)
  point P13 (43.0286, 135.0151)
  point P14 (35.2437, 148.4619)
  point P15 (54.3522, 163.3241)
  point P16 (73.4608, 144.2155)
  point P17 (68.8606, 137.1383)
  point P18 (70.276, 130)
  point P19 (275.176, 213.6284)
  point P20 (261.7086, 220.9563)
  point P21 (247.6471, 213.8265)
  point P22 (256.8536, 185.0594)
  point P23 (274.5818, 196.3981)
  point P24 (282.5038, 188.2781)
  point P25 (280, 107.7404)
  point P26 (280, 80.7669)
  point P27 (271.188, 85.0582)
  point P28 (253.1646, 77.7018)
  point P29 (263.8316, 57.1652)
  point P30 (278.1534, 60.738)
  point P31 (140, 228.0387)
  point P32 (140, 213.9426)
  point P33 (130.7001, 218.023)
  point P34 (114.7493, 220.9906)
  point P35 (109.1851, 205.0398)
  point P36 (120.1372, 191.1728)
  point P37 (134.0387, 195.0242)
  point P38 (140, 188.3471)
  point P39 (140, 92.5693)
  point P40 (130.9711, 97.1088)
  point P41 (116.5274, 95.0454)
  point P42 (108.9757, 77.3003)
  point P43 (117.7655, 63.2694)
  point P44 (133.0344, 66.5708)
  point P45 (140, 63.2694)
  point P46 (139.9962, -211.7395)
  point P47 (130.6964, -182.0636)
  point P48 (114.7456, -179.096)
  point P49 (139.9962, -172.0479)
  point P50 (139.9962, -186.144)
  point P51 (109.1813, -195.0468)
  point P52 (120.1335, -208.9138)
  point P53 (134.0349, -205.0624)
  point P54 (70.276, -270)
  point P55 (18.966, -270)
  point P56 (39.1362, -270)
  point P57 (43.0286, -264.9849)
  point P58 (35.2437, -251.5381)
  point P59 (73.4608, -255.7845)
  point P60 (54.3522, -236.6759)
  point P61 (68.8606, -262.8617)
  point P62 (70.276, -420)
  point P63 (18.966, -420)
  point P64 (39.1362, -420)
  point P65 (43.0286, -414.9849)
  point P66 (35.2437, -401.5381)
  point P67 (73.4608, -405.7845)
  point P68 (54.3522, -386.6759)
  point P69 (68.8606, -412.8617)
  point P70 (133.0344, -483.4292)
  point P71 (108.9757, -472.6997)
  point P72 (116.5274, -454.9546)
  point P73 (140, -486.7306)
  point P74 (130.9711, -452.8912)
  point P75 (117.7655, -486.7306)
  point P76 (140, -457.4307)
  point P77 (228.7481, 153.837)
  point P78 (227.6791, 130)
  point P79 (194.5419, 158.4355)
  point P80 (194.8091, 130)
  point P81 (278.1534, 60.738)
  point P82 (263.8316, 57.1652)
  point P83 (280, 107.7404)
  point P84 (280, 80.7669)
  point P85 (271.188, 85.0582)
  point P86 (253.1646, 77.7018)
  point P87 (133.0344, 66.5708)
  point P88 (108.9757, 77.3003)
  point P89 (116.5274, 95.0454)
  point P90 (140, 63.2694)
  point P91 (130.9711, 97.1088)
  point P92 (117.7655, 63.2694)
  point P93 (140, 92.5693)
  point P94 (228.7481, 153.837)
  point P95 (227.6791, 130)
  point P96 (194.5419, 158.4355)
  point P97 (194.8091, 130)
  point P98 (133.0344, 66.5708)
  point P99 (108.9757, 77.3003)
  point P100 (116.5274, 95.0454)
  point P101 (140, 63.2694)
  point P102 (130.9711, 97.1088)
  point P103 (117.7655, 63.2694)
  point P104 (140, 92.5693)
  point P105 (428.7481, -396.163)
  point P106 (427.6791, -420)
  point P107 (394.5419, -391.5645)
  point P108 (394.8091, -420)
  point P109 (478.1534, -489.262)
  point P110 (463.8316, -492.8348)
  point P111 (333.0344, -483.4292)
  point P112 (316.5274, -454.9546)
  point P113 (317.7655, -486.7306)
  point P114 (340, -457.4307)
  point P115 (308.9757, -472.6997)
  point P116 (340, -486.7306)
  point P117 (330.9711, -452.8912)
  point P118 (480, -442.2596)
  point P119 (480, -469.2331)
  point P120 (471.188, -464.9418)
  point P121 (453.1646, -472.2982)
  point P122 (340, -211.6529)
  point P123 (330.7001, -181.977)
  point P124 (314.7493, -179.0094)
  point P125 (340, -171.9613)
  point P126 (340, -186.0574)
  point P127 (309.1851, -194.9602)
  point P128 (320.1372, -208.8272)
  point P129 (334.0387, -204.9758)
  point P130 (456.8536, -214.9406)
  point P131 (461.7086, -179.0437)
  point P132 (474.5818, -203.6019)
  point P133 (482.5038, -211.7219)
  point P134 (475.176, -186.3716)
  point P135 (447.6471, -186.1735)
  point P136 (394.5419, -241.5645)
  point P137 (428.7481, -246.163)
  point P138 (427.6791, -270)
  point P139 (394.8091, -270)
  point P140 (256.8536, 185.0594)
  point P141 (261.7086, 220.9563)
  point P142 (274.5818, 196.3981)
  point P143 (282.5038, 188.2781)
  point P144 (332.4813, 139.1967)
  point P145 (328.2939, 130)
  point P146 (275.176, 213.6284)
  point P147 (247.6471, 213.8265)
  point P148 (367.3759, 146.1756)
  point P149 (336.6686, 156.8767)
  point P150 (365.0496, 130)
  point P151 (656.8536, -214.9406)
  point P152 (661.7086, -179.0437)
  point P153 (674.5818, -203.6019)
  point P154 (682.5038, -211.7219)
  point P155 (732.4813, -260.8033)
  point P156 (728.2939, -270)
  point P157 (675.176, -186.3716)
  point P158 (647.6471, -186.1735)
  point P159 (767.3759, -253.8244)
  point P160 (736.6686, -243.1233)
  point P161 (765.0496, -270)
  point P162 (678.1534, -489.262)
  point P163 (663.8316, -492.8348)
  point P164 (732.4813, -410.8033)
  point P165 (728.2939, -420)
  point P166 (767.3759, -403.8244)
  point P167 (736.6686, -393.1233)
  point P168 (765.0496, -420)
  point P169 (680, -442.2596)
  point P170 (680, -469.2331)
  point P171 (671.188, -464.9418)
  point P172 (653.1646, -472.2982)
  dimension "d3" = 420
  dimension "d4" = 260
  dimension "d5" = 140
  dimension "d6" = 140
  dimension "d7" = 130
  dimension "d8" = 140
  dimension "d9" = 20
  dimension "d10" = 20
  dimension "d11" = 20
  dimension "d12" = 20
  dimension "d13" = 20
  dimension "d14" = 20
  dimension "d16" = 140
  dimension "d17" = 20
  dimension "d18" = 20
  dimension "d19" = 1
  constraint horizontal L0
  constraint vertical L1
  constraint parallel L2 L3
  constraint perpendicular L1 L4
  constraint perpendicular L2 L5
  constraint perpendicular L0 L6
  constraint coincident L0 S6.end
  constraint coincident P0 L2
  constraint coincident P0 L5
  constraint tangent L2 A0
  constraint tangent L5 A0
  constraint tangent L0 A1
  constraint tangent L6 A1
  constraint coincident L1 S2.start
  constraint coincident origin L0
  constraint coincident origin L1
  constraint tangent L0 A2
  constraint tangent L1 A2
  constraint coincident P1 L1
  constraint coincident P1 L4
  constraint tangent L1 A3
  constraint tangent L4 A3
  constraint vertical L8
  constraint perpendicular L7 L8
  constraint tangent A4 L8
  constraint tangent L7 A4
  constraint horizontal L10
  constraint vertical L9
  constraint tangent A5 L10
  constraint tangent L9 A5
  constraint horizontal L11
  constraint coincident S6.end L11
  constraint horizontal L12
  constraint coincident S6.end L12
  constraint coincident L0 S4.end
  constraint horizontal L13
  constraint perpendicular L15 L16
  constraint perpendicular L17 L18
  constraint tangent A6 L18
  constraint tangent A6 L17
  constraint tangent A7 L19
  constraint horizontal L20
  measures "d3" distance of P0 P1
  measures "d4" distance of origin P1
  measures "d5" distance of P0 L2.end
  measures "d8" distance of L2.end L3.end
  measures "d7" distance of P0 L5.end
  measures "d8" distance of P1 L3.end A1.centre
  measures "d9" radius of A0
  measures "d10" radius of A1
  measures "d11" radius of A2
  measures "d12" radius of A3
  measures "d13" radius of A4
  measures "d14" radius of A5
  measures "d16" distance of S19.start L14.end
  measures "d17" radius of A6
  measures "d18" radius of A7
extrude "Extrude1" add sketch "Sketch1" along normal blind 20 contours L7 A4 L8 S7 S8 | S9 S10 L9 A5 L10 | L13 S16 S17 S18 | S19 L14 S20 S21 | A6 L17 S24 S25 L18 | A7 L19 S26 S27 L20 makes body 1 at (750.5808, -491.2587, 0) makes body 2 at (60.3337, -188.2155, 0) makes body 3 at (425.9828, -529.7692, 0) makes body 4 at (741.849, -186.0979, 0) makes body 5 at (396.4237, -204.111, 0) makes body 6 at (48.3818, -475.3441, 0)
move_body "Move1" [rolled back]
move_body "Move2" [rolled back]
move_body "Move3" [rolled back]
equation "lengd = 420 mm"
equation "Breidd = 260 mm"
equation "d5 = lengd / 3"
equation "d6 = lengd / 3"
equation "d7 = Breidd / 2"
equation "d16 = lengd / 3"
